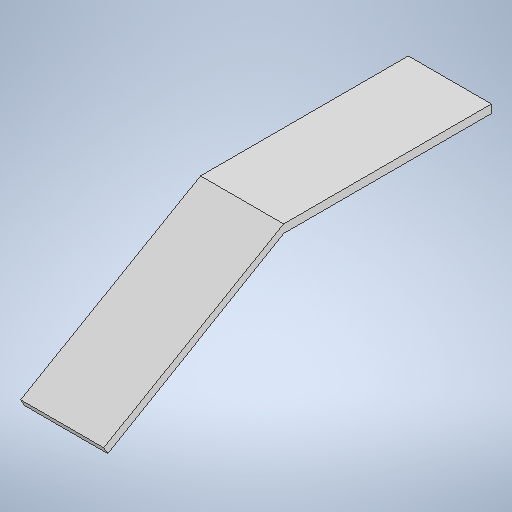
# Autodesk Inventor part: extended150degreebracket
Saved by Autodesk Inventor 2025.2 (Build 292293000, 293)
## iProperties
Created: 2026-03-28
Part Number: extended150degreebracket
Material: Generic
Document SubType Name: Modeling
Designer: hp
Density: 1 g/cm^3
Appearance: Default
Author: hp
Autodesk Inventor part; units mm, degrees
ref_plane "YZ Plane" through (0, 0, 0) normal (1, 0, 0) x (0, 1, 0)
ref_plane "XZ Plane" through (0, 0, 0) normal (0, 1, 0) x (-1, 0, 0)
ref_plane "XY Plane" through (0, 0, 0) normal (0, 0, 1) x (1, 0, 0)
sketch "Sketch1" plane through (0, 0, 0) normal (1, 0, 0) x (0, 1, 0)
  line L0 (0, 0) -> (0, -50)
  line L1 (0, -50) -> (2, -50)
  line L2 (2, -50) -> (2, 0)
  line L3 (2, 0) -> (-23, 43.3013)
  line L4 (-23, 43.3013) -> (-24.7321, 42.3013)
  line L5 (-24.7321, 42.3013) -> (0, 0)
  dimension "d0" = 50
  dimension "d1" = 2
  dimension "d2" = 50
  dimension "d3" = 150
  dimension "d4" = 2
  constraints: 12 end point, 3 perpendicular, 1 vertical
  measures "d0" distance of L0.start L0.end
  measures "d1" distance of L0.end L1.end
  measures "d2" distance of L2.end L3.end
  measures "d3" angle of L3 L2
  measures "d4" distance of L3.end L4.end
extrude "Extrusion1" add sketch "Sketch1" against normal blind 20
body "Solid1"
